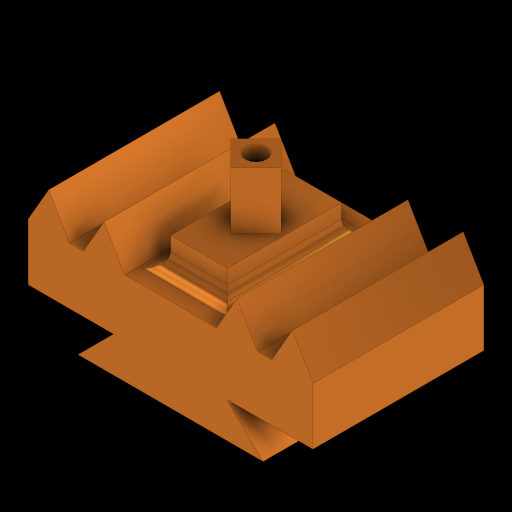
# Autodesk Inventor part: 2020-10-BK
Saved by Autodesk Inventor 2024 (Build 280153000, 153)
## iProperties
Created: 2023-10-27
Part Number: 2020-10-BK
Material: Gold
Document SubType Name: Modeling
Designer: bennk
Mass: 7514.63 g
Surface Area: 497.749 cm^2
Volume: 389.359 cm^3
Density: 19.3 g/cm^3
Appearance: Metal 1600F Hot
Author: bennk
Autodesk Inventor part; units mm, degrees
ref_plane "YZ Plane" through (0, 0, 0) normal (1, 0, 0) x (0, 1, 0)
ref_plane "XZ Plane" through (0, 0, 0) normal (0, 1, 0) x (-1, 0, 0)
ref_plane "XY Plane" through (0, 0, 0) normal (0, 0, 1) x (1, 0, 0)
sketch "Sketch1" plane through (0, 0, 0) normal (0, 0, 1) x (1, 0, 0)
  line L0 (0, 0) -> (0, 25.4)
  line L1 (0, 25.4) -> (9.1654, 41.275)
  line L2 (9.1654, 41.275) -> (18.3309, 25.4)
  line L3 (18.3309, 25.4) -> (24.6809, 25.4)
  line L4 (24.6809, 25.4) -> (33.8463, 41.275)
  line L5 (33.8463, 41.275) -> (43.0117, 25.4)
  line L6 (43.0117, 25.4) -> (83.9883, 25.4)
  line L7 (102.3191, 25.4) -> (108.6691, 25.4)
  line L8 (108.6691, 25.4) -> (117.8346, 41.275)
  line L9 (117.8346, 41.275) -> (127, 25.4)
  line L10 (127, 25.4) -> (127, 0)
  line L11 (127, 0) -> (88.9, 0)
  line L12 (88.9, 0) -> (104.775, -15.875)
  line L13 (104.775, -15.875) -> (22.225, -15.875)
  line L14 (22.225, -15.875) -> (38.1, 0)
  line L15 (38.1, 0) -> (0, 0)
  line L16 (9.1654, 41.275) -> (117.8346, 41.275) construction
  line L17 (102.3191, 25.4) -> (93.1537, 41.275)
  line L18 (83.9883, 25.4) -> (93.1537, 41.275)
  dimension "d0" = 45
  dimension "d1" = 45
  dimension "d2" = 127
  dimension "d3" = 60
  dimension "d4" = 6.35
  dimension "d5" = 25.4
  dimension "d6" = 25.4
  dimension "d7" = 38.1
  dimension "d8" = 15.875
  dimension "d9" = 6.35
  dimension "d10" = 60
  dimension "d12" = 60
  dimension "d13" = 25.4
  dimension "d14" = 25.4
  dimension "d15" = 25.4
  dimension "d16" = 15.875
  dimension "d17" = 60
  constraints: 39 end point, 5 equal length, 5 horizontal, 2 point on line, 2 vertical, 1 collinear, 1 perpendicular
  measures "d0" angle of L15 L14
  measures "d1" angle of L11 L12
  measures "d2" distance between parallel lines of L0 L10
  measures "d3" angle of L2 L1
  measures "d4" distance of L3.end L2.end
  measures "d5" distance of L0.start L0.end
  measures "d6" distance of L9.end L10.end
  measures "d7" distance of L10.end L11.end
  measures "d8" distance between parallel lines of L11 L13
  measures "d9" distance of L7.end L7.start
  measures "d10" angle of L5 L4
  measures "d12" angle of L9 L8
  measures "d13" distance between parallel lines of L11 L7
  measures "d14" distance between parallel lines of L15 L6
  measures "d15" distance between parallel lines of L15 L3
  measures "d16" vertical distance of L1.end L0.end
  measures "d17" angle of L17 L18
extrude "MAIN BODY" add sketch "Sketch1" along normal mid plane 76.2
sketch "Sketch2" plane through (43.0117, 25.4, 38.1) normal (0, 1, 0) x (1, 0, 0)
  line L0 (7.7883, 12.7) -> (33.1883, 12.7)
  line L1 (33.1883, 12.7) -> (33.1883, 63.5)
  line L2 (33.1883, 63.5) -> (7.7883, 63.5)
  line L3 (7.7883, 63.5) -> (7.7883, 12.7)
  line L4 (40.9765, 0) -> (0, 0) projected
  line L5 (0, 76.2) -> (40.9765, 76.2) projected
  line L6 (40.9765, 76.2) -> (40.9765, 0) projected
  line L7 (0, 76.2) -> (0, 0) projected
  point P0 (-43.0117, 38.1)
  point P1 (20.4883, 12.7)
  dimension "d25" = 50.8
  dimension "d26" = 25.4
  dimension "d27" = 12.7
  dimension "d28" = 40.9765
  dimension "d29" = 7.7883
  dimension "d30" = 76.2
  constraints: 8 end point, 2 parallel, 1 horizontal, 1 midpoint, 1 perpendicular
  measures "d25" distance of L0.end L1.end
  measures "d26" distance of L0.start L0.end
  measures "d27" distance from line of L4 point (20.488, 12.7)
  measures "d28" distance between parallel lines of L6 L7
  measures "d29" distance between parallel lines of L6 L1
  measures "d30" distance between parallel lines of L5 L4
extrude "LARGE BOSS" add sketch "Sketch2" along normal blind 12.7 contours L3 L2 L1 L0
sketch "Sketch3" plane through (43.0117, 38.1, 38.1) normal (0, 1, 0) x (1, 0, 0)
  line L0 (7.7883, 12.7) -> (7.7883, 63.5) projected
  line L1 (9.2629, 38.1) -> (20.4883, 26.8747)
  line L2 (20.4883, 26.8747) -> (31.7136, 38.1)
  line L3 (31.7136, 38.1) -> (20.4883, 49.3253)
  line L4 (20.4883, 49.3253) -> (9.2629, 38.1)
  line L5 (33.1883, 12.7) -> (33.1883, 63.5) projected
  line L6 (7.7883, 63.5) -> (33.1883, 63.5) projected
  line L7 (20.4883, 63.5) -> (20.4883, 12.7) construction
  line L8 (7.7883, 12.7) -> (33.1883, 12.7) projected
  line L9 (7.7883, 38.1) -> (33.1883, 38.1) construction
  point P0 (-43.0117, 38.1)
  dimension "d34" = 15.875
  dimension "d35" = 15.875
  dimension "d36" = 45
  constraints: 12 end point, 4 midpoint, 4 point on line, 2 parallel, 1 perpendicular
  measures "d34" distance of L1.start L1.end
  measures "d35" distance of L2.end L1.end
  measures "d36" angle of L0 L1
extrude "TALL BOSS" add sketch "Sketch3" along normal blind 25.4 contours L4 L3 L2 L1
sketch "Sketch4" plane through (43.0117, 63.5, 38.1) normal (0, 1, 0) x (1, 0, 0)
  line L0 (20.4883, 49.3253) -> (9.2629, 38.1) projected
  line L1 (20.4883, 26.8747) -> (31.7136, 38.1) projected
  line L2 (9.2629, 38.1) -> (31.7136, 38.1)
  line L3 (31.7136, 38.1) -> (20.4883, 49.3253) projected
  line L4 (20.4883, 49.3253) -> (20.4883, 26.8747)
  point P0 (-43.0117, 38.1)
  point P1 (20.4883, 38.1)
  constraints: 4 end point, 1 horizontal, 1 midpoint, 1 point on line, 1 vertical
hole "THROUGH HOLE" at (63.5, 63.5, 0) direction (0, -1, 0) diameter 9.525 end through all
fillet "LARGE BOSS FILLET" radius 6.35 4 edges at (76.2, 25.4, 0) (63.5, 25.4, -25.4) (50.8, 25.4, 0) (63.5, 25.4, 25.4)
equation "\"d1\" = d0"
equation "\"d6\" = d5"
equation "\"d9\" = d4"
equation "\"d10\" = d3"
equation "\"d12\" = d11"
equation "\"d13\" = d6"
equation "\"d14\" = d13"
equation "\"d27\" = -0.5 * d25 + 0.5 * d30"
equation "\"d29\" = -0.5 * d26 + 0.5 * d28"
equation "\"d11\" = d10"
body "Solid1"
